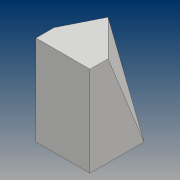
# Autodesk Inventor part: 40
Saved by Autodesk Inventor 2018 (Build 220112000, 112)
## iProperties
Created: 2020-09-18
Part Number: 40
Material: 一般
Document SubType Name: Modeling
Designer: 88697
Density: 1 g/cm^3
Appearance: 預設
Author: 88697
Autodesk Inventor part; units mm, degrees
ref_plane "YZ Plane" through (0, 0, 0) normal (1, 0, 0) x (0, 1, 0)
sketch "草圖1" plane through (0, 0, 0) normal (0, 1, 0) x (-1, 0, 0)
  line L0 (0, 0) -> (-30, 0)
  line L1 (-30, 0) -> (-30, -50)
  line L2 (-30, -50) -> (0, -50)
  line L3 (0, -50) -> (0, 0)
  dimension "d0" = 30
  dimension "d1" = 50
  constraints: 8 end point, 2 parallel, 1 horizontal, 1 perpendicular
  measures "d0" distance of L0.start L0.end
  measures "d1" distance of L2.end L0.start
extrude "擠出1" add sketch "草圖1" along normal blind 30
sketch "草圖2" plane through (0, 0, 0) normal (0, 0, 1) x (1, 0, 0)
  line L0 (0, 0) -> (0, 30) projected
  line L1 (30, 0) -> (30, 30) projected
  line L2 (0, 0) -> (30, 0) projected
  line L3 (0, 30) -> (30, 30) projected
  point P0 (0, 10)
  point P1 (30, 10)
  point P2 (10, 30)
  dimension "d4" = 10
  dimension "d5" = 10
  dimension "d6" = 10
  constraints: 3 point on line
  measures "d4" distance from line of L2 point (0, 10)
  measures "d5" distance from line of L2 point (30, 10)
  measures "d6" distance from line of L0 point (10, 30)
ref_plane "工作平面1" through (0, 30, -50) normal (0.8805, -0.4402, -0.1761) x (0.1961, 0, 0.9806)
sketch "草圖3" plane through (0, 30, -50) normal (0.8805, -0.4402, -0.1761) x (0.1961, 0, 0.9806)
  line L0 (-9.0591, -8.5092) -> (64.1783, -8.5092)
  line L1 (64.1783, -8.5092) -> (64.1783, 25.3878)
  line L2 (64.1783, 25.3878) -> (-9.0591, 25.3878)
  line L3 (-9.0591, 25.3878) -> (-9.0591, -8.5092)
  point P0 (49.029, 31.2534)
  constraints: 8 end point, 2 parallel, 1 horizontal, 1 perpendicular
extrude "擠出2" cut sketch "草圖3" against normal blind 30
ref_plane "工作平面2" through (30, 30, -50) normal (0.6804, 0.6804, 0.2722) x (-0.3714, 0, 0.9285)
sketch "草圖4" plane through (30, 30, -50) normal (0.6804, 0.6804, 0.2722) x (-0.3714, 0, 0.9285)
  line L0 (68.88, -9.2139) -> (-15.4545, -9.2139)
  line L1 (-15.4545, -9.2139) -> (-15.4545, 38.1391)
  line L2 (-15.4545, 38.1391) -> (68.88, 38.1391)
  line L3 (68.88, 38.1391) -> (68.88, -9.2139)
  point P0 (57.5656, 15.6674)
  constraints: 8 end point, 2 parallel, 1 horizontal, 1 perpendicular
extrude "擠出3" cut sketch "草圖4" along normal blind 30
